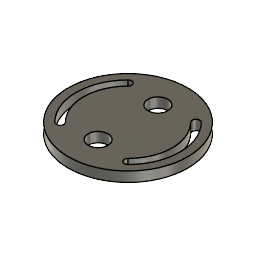
valvefixed0506_v0.1 (Autodesk Fusion 360 design; units mm, degrees)
Autodesk Fusion 360 part; units mm, degrees
sketch "Sketch1" plane through (0, 0, 0) normal (0, 0, 1) x (1, 0, 0)
  circle A0 centre (0, -15) radius 5
  circle A1 centre (0, 15) radius 5
  line L0 (26.5, 0) -> (27.807, 0) construction
  circle A2 centre (0, 0) radius 30
  line L1 (22.25, 0) -> (27.7377, 0) construction
  arc A3 (18.3848, 18.3848) -> (15.7331, 15.7331) centre (17.059, 17.059) ccw
  arc A4 (-15.7331, 15.7331) -> (-18.3848, 18.3848) centre (-17.059, 17.059) ccw
  arc A5 (15.7331, -15.7331) -> (18.3848, -18.3848) centre (17.059, -17.059) ccw
  arc A6 (-18.3848, -18.3848) -> (-15.7331, -15.7331) centre (-17.059, -17.059) ccw
  arc A7 (-15.7331, 15.7331) -> (-15.7331, -15.7331) centre (0, 0) ccw
  arc A8 (15.7331, -15.7331) -> (15.7331, 15.7331) centre (0, 0) ccw
  arc A9 (-18.3848, 18.3848) -> (-18.3848, -18.3848) centre (0, 0) ccw
  arc A10 (18.3848, -18.3848) -> (18.3848, 18.3848) centre (0, 0) ccw
  dimension "d4" = 15
  dimension "d5" = 10
  dimension "d11" = 60
  dimension "d12" = 52
  dimension "d16" = 44.5
  dimension "d17" = 3.75
  constraint coincident A2.centre A7.centre
  constraint horizontal L1
  constraint symmetric L1 A3.end A5.start
  constraint symmetric L1 A3.start A5.end
  constraint symmetric L1 A3 A5
  constraint symmetric L1 A4.end A6.start
  constraint symmetric L1 A4.start A6.end
  constraint symmetric L1 A4 A6
  constraint coincident L1.start A8
  constraint concentric A7 A8
  constraint concentric A9 A10
  measures "d4" distance of A2.centre A1.centre
  measures "d5" diameter of A1
  measures "d11" diameter of A2
  measures "d12" diameter of A9
  measures "d16" diameter of A7
  measures "d17" diameter of A3
extrude "Extrude1" add sketch "Sketch1" along normal blind 5
